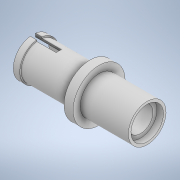
# Autodesk Inventor part: VasileAxle
Saved by Autodesk Inventor 2020 (Build 240168000, 168)
## iProperties
Created: 2020-02-14
Part Number: VasileAxle
Material: Generic
Document SubType Name: Modeling
Designer: al
Density: 1 g/cm^3
Appearance: Default
Author: al
Autodesk Inventor part; units mm, degrees
ref_plane "YZ Plane" through (0, 0, 0) normal (1, 0, 0) x (0, 1, 0)
ref_plane "XZ Plane" through (0, 0, 0) normal (0, 1, 0) x (-1, 0, 0)
ref_plane "XY Plane" through (0, 0, 0) normal (0, 0, 1) x (1, 0, 0)
sketch "Sketch2" plane through (0, 0, 0) normal (0, 0, 1) x (1, 0, 0)
  line L0 (-0.4505, 4.5581) -> (1.3275, 4.5581)
  line L1 (1.0735, -0.5219) -> (1.0735, 1.8911)
  line L2 (-0.4505, -0.5219) -> (1.0735, -0.5219)
  line L3 (1.0735, 1.8911) -> (9.4555, 1.8911)
  line L4 (9.4555, 1.8911) -> (9.4555, 2.6531)
  line L5 (9.4555, 2.6531) -> (10.7255, 2.6531)
  line L6 (10.7255, 2.6531) -> (10.7255, 3.1611)
  line L7 (10.7255, 3.1611) -> (1.3275, 3.1611)
  line L8 (1.3275, 3.1611) -> (1.3275, 4.5581)
  line L9 (-0.4505, 1.8911) -> (-5.2765, 1.8911)
  line L10 (-5.2765, 1.8911) -> (-5.2765, 2.6531)
  line L11 (-5.2765, 2.6531) -> (-11.6265, 2.6531)
  line L12 (-11.6265, 2.6531) -> (-11.6265, 3.2881)
  line L13 (-11.6265, 3.2881) -> (-10.3565, 3.2881)
  line L14 (-10.3565, 3.2881) -> (-10.3565, 3.0341)
  line L15 (-10.3565, 3.0341) -> (-0.4505, 3.0341)
  line L16 (-0.4505, 4.5581) -> (-0.4505, 3.0341)
  line L17 (-0.4505, 1.8911) -> (-0.4505, -0.5219)
  point P0 (0, 0)
  dimension "d2" = 2.413
  dimension "d4" = 8.382
  dimension "d5" = 0.762
  dimension "d6" = 90
  dimension "d7" = 1.27
  dimension "d8" = 0.508
  dimension "d9" = 4.826
  dimension "d10" = 0
  dimension "d11" = 0.762
  dimension "d12" = 6.35
  dimension "d13" = 0.635
  dimension "d14" = 1.27
  dimension "d15" = 0.254
  constraints: 36 end point, 7 horizontal, 5 perpendicular, 4 vertical, 1 collinear
  measures "d2" distance of L1.start L1.end
  measures "d4" distance of L1.end L3.end
  measures "d5" distance of L3.end L4.end
  measures "d6" angle of L4 L3
  measures "d7" distance of L4.end L5.end
  measures "d8" distance of L5.end L6.end
  measures "d9" distance of L9.start L9.end
  measures "d10" distance between parallel lines of L3 L9
  measures "d11" distance of L9.end L10.end
  measures "d12" distance of L10.end L11.end
  measures "d13" distance of L11.end L12.end
  measures "d14" distance of L12.end L13.end
  measures "d15" distance of L13.end L14.end
revolve "Revolution1" add sketch "Sketch2" angle 360 mid plane about axis through (-0.4505, -0.5219, 0) along (1, 0, 0)
sketch "Sketch3" plane through (-11.6265, -0.5219, 0) normal (-1, 0, 0) x (0, 0, 1)
  line L0 (-0.508, 6.3203) -> (0.508, 6.3203)
  line L1 (0.508, 6.3203) -> (0.508, -5.6235)
  line L2 (0.508, -5.6235) -> (-0.508, -5.6235)
  line L3 (-0.508, -5.6235) -> (-0.508, 6.3203)
  point P0 (0, 0.5219)
  dimension "d17" = 1.016
  dimension "d18" = 0.508
  constraints: 8 end point, 2 parallel, 1 horizontal, 1 perpendicular
  measures "d17" distance of L1.end L2.end
  measures "d18" distance from line of L1 point (0, 0.522)
extrude "Extrusion1" cut sketch "Sketch3" against normal blind 5.08
body "Solid1"
